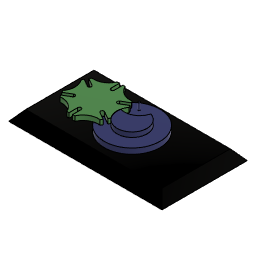
Geneva mechanism (Autodesk Fusion 360 design; units mm, degrees)
Autodesk Fusion 360 part; units mm, degrees
sketch "lower platform" plane through (0, 0, 0) normal (0, 0, 1) x (1, 0, 0) in component "Platform"
  line L0 (-112.5, 62.5) -> (112.5, 62.5)
  line L1 (112.5, 62.5) -> (112.5, -62.5)
  line L2 (112.5, -62.5) -> (-112.5, -62.5)
  line L3 (-112.5, -62.5) -> (-112.5, 62.5)
  line L4 (-112.5, 62.5) -> (112.5, -62.5) construction
  line L5 (112.5, 62.5) -> (-112.5, -62.5) construction
  dimension "d1" = 225
  dimension "d2" = 125
  constraint horizontal L0
  constraint perpendicular L0 L1
  constraint parallel L0 L2
  constraint parallel L1 L3
  constraint coincident L4 origin
  constraint coincident L5 origin
  measures "d1" distance of L1.end L2.end
  measures "d2" distance of L0.end L1.end
ref_plane "WorkPlane1" through (0, 0, 15) normal (0, 0, 1) x (1, 0, 0) in component "Platform"
sketch "upper platform" plane through (0, 0, 15) normal (0, 0, 1) x (1, 0, 0) in component "Platform"
  line L0 (-100, 50) -> (100, 50)
  line L1 (100, 50) -> (100, -50)
  line L2 (100, -50) -> (-100, -50)
  line L3 (-100, -50) -> (-100, 50)
  line L4 (-100, 50) -> (100, -50) construction
  line L5 (100, 50) -> (-100, -50) construction
  dimension "d4" = 200
  dimension "d5" = 100
  constraint horizontal L0
  constraint perpendicular L0 L1
  constraint parallel L0 L2
  constraint parallel L1 L3
  constraint coincident L4 origin
  constraint coincident L5 origin
  measures "d4" distance of L1.end L2.end
  measures "d5" distance of L0.end L1.end
loft "Loft1" add profiles "lower platform", "upper platform" section 1 section 2 makes body 1 in component "Platform"
sketch "snowflake" plane through (0, 0, 15) normal (0, 0, 1) x (-1, 0, 0) in component "Snowflake"
  line L0 (100, 50) -> (-100, 50)
  line L1 (-100, 50) -> (-100, -50)
  line L2 (-100, -50) -> (100, -50)
  line L3 (100, -50) -> (100, 50)
  circle A0 centre (47, 0) radius 4.5
  line L4 (47, 0) -> (47, -4.5)
  line L5 (44.5078, -24.6971) -> (44.5078, -37.4171)
  line L6 (49.4922, -24.6971) -> (49.4922, -37.4171)
  arc A1 (49.4922, -24.6971) -> (44.5078, -24.6971) centre (47, -24.5) ccw
  line L7 (69.6345, -10.1902) -> (80.6503, -16.5502)
  arc A2 (69.6345, -10.1902) -> (67.1422, -14.5069) centre (68.2176, -12.25) ccw
  line L8 (67.1422, -14.5069) -> (78.158, -20.8669)
  line L9 (67.1422, 14.5069) -> (78.158, 20.8669)
  arc A3 (67.1422, 14.5069) -> (69.6345, 10.1902) centre (68.2176, 12.25) ccw
  line L10 (69.6345, 10.1902) -> (80.6503, 16.5502)
  line L11 (44.5078, 24.6971) -> (44.5078, 37.4171)
  arc A4 (44.5078, 24.6971) -> (49.4922, 24.6971) centre (47, 24.5) ccw
  line L12 (49.4922, 24.6971) -> (49.4922, 37.4171)
  line L13 (24.3655, 10.1902) -> (13.3497, 16.5502)
  arc A5 (24.3655, 10.1902) -> (26.8578, 14.5069) centre (25.7824, 12.25) ccw
  line L14 (26.8578, 14.5069) -> (15.842, 20.8669)
  line L15 (26.8578, -14.5069) -> (15.842, -20.8669)
  arc A6 (26.8578, -14.5069) -> (24.3655, -10.1902) centre (25.7824, -12.25) ccw
  line L16 (24.3655, -10.1902) -> (13.3497, -16.5502)
  arc A7 (82.0355, 13.3702) -> (82.0355, -13.3702) centre (100, 0) ccw
  arc A8 (52.9388, 37.0268) -> (76.0967, 23.6565) centre (73.5, 45.8993) ccw
  arc A9 (17.9033, 23.6565) -> (41.0612, 37.0268) centre (20.5, 45.8993) ccw
  arc A10 (11.9645, -13.3702) -> (11.9645, 13.3702) centre (-6, 0) ccw
  arc A11 (41.0612, -37.0268) -> (17.9033, -23.6565) centre (20.5, -45.8993) ccw
  arc A12 (76.0967, -23.6565) -> (52.9388, -37.0268) centre (73.5, -45.8993) ccw
  arc A13 (41.0612, -37.0268) -> (52.9388, -37.0268) centre (47, 0) ccw
  arc A14 (15.842, -20.8669) -> (17.9033, -23.6565) centre (47, 0) ccw
  arc A15 (11.9645, -13.3702) -> (13.3497, -16.5502) centre (47, 0) ccw
  arc A16 (13.3497, 16.5502) -> (11.9645, 13.3702) centre (47, 0) ccw
  arc A17 (17.9033, 23.6565) -> (15.842, 20.8669) centre (47, 0) ccw
  arc A18 (44.5078, 37.4171) -> (41.0612, 37.0268) centre (47, 0) ccw
  arc A19 (52.9388, 37.0268) -> (49.4922, 37.4171) centre (47, 0) ccw
  arc A20 (78.158, 20.8669) -> (76.0967, 23.6565) centre (47, 0) ccw
  arc A21 (82.0355, 13.3702) -> (80.6503, 16.5502) centre (47, 0) ccw
  arc A22 (76.0967, -23.6565) -> (78.158, -20.8669) centre (47, 0) ccw
  arc A23 (80.6503, -16.5502) -> (82.0355, -13.3702) centre (47, 0) ccw
  dimension "d6" = 75
  dimension "d7" = 9
  dimension "d8" = 5
  dimension "d11" = 360
  dimension "d14" = 360
  constraint concentric A0 A22
  constraint coincident A0.centre L4.start
  constraint perpendicular L2 L4
  constraint coincident L4 A1.centre
  constraint coincident L5.end A22
  constraint parallel L4 L5
  constraint coincident L6.end A22
  constraint parallel L4 L6
  constraint coincident A0 L4.end
  constraint midpoint L3 A7.centre
  constraint coincident A7.start A22
  constraint concentric A13 A22
  constraint concentric A14 A22
  constraint concentric A15 A22
  constraint concentric A16 A22
  constraint concentric A17 A22
  constraint concentric A18 A22
  constraint concentric A19 A22
  constraint concentric A20 A22
  constraint concentric A21 A22
  constraint concentric A22 A23
  measures "d6" diameter of A22
  measures "d7" diameter of A0
  measures "d8" diameter of A1
extrude "Extrude1" add sketch "snowflake" along normal blind 7 separate body contours L5 L6 A1 L7 A2 L8 L9 A3 L10 L11 A4 L12 L13 A5 L14 L15 A6 L16 A7 A8 A9 A10 A11 A12 A13 A14 A15 A16 A17 A18 A19 A20 A21 A22 A23 makes body 2 in component "Snowflake"
extrude "Extrude2" add sketch "snowflake" along normal blind 15 separate body contours A0 makes body 3 in component "Snowflake"
move_body "Align1" bodies 2 to x (1, 0, 0) y (0, 1, 0) z (0, 0, 1) at (0, 0, 8) in component "Snowflake"
sketch "crank" plane through (0, 0, 15) normal (0, 0, 1) x (-1, 0, 0) in component "Crank"
  line L0 (100, 50) -> (-100, 50)
  line L1 (-100, 50) -> (-100, -50)
  line L2 (-100, -50) -> (100, -50)
  line L3 (100, -50) -> (100, 50)
  circle A0 centre (-6, 0) radius 22
  arc A1 (9.0666, 16.0864) -> (9.1411, -15.9608) centre (24.8992, 0.0995) ccw
  circle A2 centre (-6, 0) radius 41
  dimension "d19" = 22.5
  dimension "d22" = 82
  constraint coincident A0 A1.end
  constraint concentric A0 A2
  measures "d19" radius of A1
  measures "d22" diameter of A2
extrude "Extrude2'" add sketch "crank" along normal blind 8 separate body contours A2 makes body 4 in component "Crank"
extrude "Extrude1'" add sketch "crank" along normal blind 7 separate body contours A0 A1 picked at (-7.6949, -0.0055) makes body 5 in component "Crank"
extrude "Extrude3" add sketch "crank" along normal blind 8 contours A0 A1 | A0 A1 bodies 4 in component "Crank"
move_body "Align1'" bodies 5 to x (1, 0, 0) y (0, 1, 0) z (0, 0, 1) at (0, 0, 8) in component "Crank"
combine "Combine1" operation add target body 4 tool bodies 5 in component "Crank"
sketch "Sketch2" plane through (0, 0, 23) normal (0, 0, 1) x (-1, 0, 0) in component "Crank"
  arc A0 (9.038, 16.058) -> (9.1411, -15.9608) centre (24.8992, 0.0995) ccw
  arc A1 (9.038, 16.058) -> (9.1411, -15.9608) centre (-6, 0) ccw
  circle A2 centre (-6, 0) radius 41
  circle A3 centre (20.5, 0) radius 1.5
  dimension "d32" = 3
  measures "d32" diameter of A3
extrude "Extrude4" add sketch "Sketch2" along normal blind 10 contours A3 bodies 4 in component "Crank"
move_face "MoveFace1" to x (1, 0, 0) y (0, 1, 0) z (0, 0, 1) at (-1, 0, 0) 2 faces at (-20.3514, -0.9861, 33) (-21.9981, 0.0748, 29.6667) on bodies 4 in component "Crank"
move_face "MoveFace2" to x (1, 0, 0) y (0, 1, 0) z (0, 0, 1) at (-1, 0, 0) 2 faces at (-22.9981, 0.0748, 29.6667) (-21.1335, 0.6348, 33) on bodies 4 in component "Crank"
combine "Combine1'" operation add target body 2 tool bodies 3 in component "Snowflake"
component "Platform" placed x (1, 0, 0) y (0, 1, 0) z (0, 0, 1) at (0, 0, 0)
component "Crank" placed x (0.886204, -0.463296, 0) y (0.463296, 0.886204, 0) z (0, 0, 1) at (0.6828, 2.7798, 0)
component "Snowflake" placed x (0.998891, -0.047072, 0) y (0.047072, 0.998891, 0) z (0, 0, 1) at (-0.0521, -2.2124, 0)
named bodies: "platform", "snowflake", "snowflake base", "crank"
